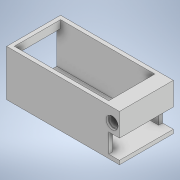
# Autodesk Inventor part: chaimber
Saved by Autodesk Inventor 2021 (Build 250183000, 183)
## iProperties
Created: 2024-03-14
Part Number: chaimber
Material: Generic
Document SubType Name: Modeling
Designer: 22hamfri
Density: 1 g/cm^3
Appearance: Default
Author: 22hamfri
Autodesk Inventor part; units mm, degrees
ref_plane "YZ Plane" through (0, 0, 0) normal (1, 0, 0) x (0, 1, 0)
ref_plane "XZ Plane" through (0, 0, 0) normal (0, 1, 0) x (-1, 0, 0)
ref_plane "XY Plane" through (0, 0, 0) normal (0, 0, 1) x (1, 0, 0)
sketch "Sketch1" plane through (0, 0, 0) normal (0, 1, 0) x (-1, 0, 0)
  line L0 (-24.5, 12) -> (24.5, 12)
  line L1 (24.5, 12) -> (24.5, -12)
  line L2 (24.5, -12) -> (-24.5, -12)
  line L3 (-24.5, -12) -> (-24.5, 12)
  line L4 (-24.5, 12) -> (24.5, -12) construction
  line L5 (24.5, 12) -> (-24.5, -12) construction
  line L6 (26.5, 14) -> (26.5, -14)
  line L7 (-24.5, 12) -> (-24.5, 14)
  line L8 (-24.5, 14) -> (26.5, 14)
  line L9 (26.5, -14) -> (-24.5, -14)
  line L10 (-24.5, -14) -> (-24.5, -12)
  line L11 (24.5, 12) -> (26.5, 12)
  line L12 (24.5, -12) -> (26.5, -12)
  point P0 (0, 0)
  dimension "d0" = 24
  dimension "d1" = 49
  dimension "d2" = 2
  dimension "d3" = 2
  dimension "d4" = 2
  constraints: 26 end point, 5 perpendicular, 2 horizontal, 2 midpoint, 2 parallel, 2 point on line, 2 vertical
  measures "d0" distance between parallel lines of L2 L0
  measures "d1" distance between parallel lines of L1 L3
  measures "d2" distance between parallel lines of L6 L1
  measures "d3" distance between parallel lines of L9 L2
  measures "d4" distance between parallel lines of L0 L8
extrude "Extrusion1" add sketch "Sketch1" against normal blind 2
extrude "Extrusion2" add sketch "Sketch1" along normal blind 22 contours L7 L8 L6 L11 L0 | L2 L12 L6 L9 L10
sketch "Sketch2" plane through (-26.5, 0, -12) normal (0, 0, 1) x (1, 0, 0)
  line L0 (0, 22) -> (0, 20)
  line L1 (0, 0) -> (0, 22) projected
  line L2 (0, 22) -> (2, 22)
  line L3 (0, 22) -> (51, 22) projected
  line L4 (2, 22) -> (2, 18)
  arc A0 (2, 18) -> (0, 20) centre (-3.1231, 14.8769) ccw
  line L5 (51, 0) -> (0, 0) projected
  point P0 (26.5, 0)
  dimension "d13" = 18
  dimension "d14" = 20
  dimension "d15" = 2
  dimension "d16" = 6
  constraints: 6 end point, 2 point on circle, 2 point on line, 1 centre point, 1 vertical
  measures "d13" distance from line of L5 L4.end
  measures "d14" distance from line of L5 L0.end
  measures "d15" distance between parallel lines of L1 L4
  measures "d16" radius of A0
extrude "Extrusion3" add sketch "Sketch2" along normal up to surface (24 mm away)
sketch "Sketch4" plane through (-26.5, -2, 14) normal (0, 0, 1) x (1, 0, 0)
  circle A0 centre (54.8, 17) radius 2.575
  circle A1 centre (54.8, 17) radius 3.1
  circle A2 centre (54.8, 17) radius 3.8
  line L0 (51, 2) -> (51, 24) projected
  line L1 (51, 12) -> (58.6, 12)
  line L2 (58.6, 12) -> (58.6, 24)
  line L3 (58.6, 24) -> (51, 24)
  point P0 (26.5, 2)
  dimension "d31" = 5.15
  dimension "d32" = 6.2
  dimension "d33" = 0.7
  dimension "d34" = 10
  dimension "d35" = 15
  constraints: 6 end point, 3 centre point, 3 perpendicular, 2 tangent, 1 point on line
  measures "d31" diameter of A0
  measures "d32" diameter of A1
  measures "d33" radial gap between concentric circles of A1 A2
  measures "d34" distance from line of L0.start L1
  measures "d35" vertical distance of L0.start A0.centre
extrude "Extrusion4" add sketch "Sketch4" against normal up to surface (28 mm away) contours A1 | A2 | L2 L1 L0 A2 | A2 L0 L3 L2
extrude "Extrusion5" cut sketch "Sketch4" against normal blind 1 contours A1
sketch "Sketch5" plane through (24.5, -2, 14) normal (1, 0, 0) x (0, 0, -1)
  line L0 (0, 0) -> (0, 12) projected
  line L1 (0, 2) -> (28, 2)
  line L2 (28, 0) -> (28, 12) projected
  line L3 (2, 2) -> (26, 2) projected
  line L4 (28, 12) -> (26, 12) projected
  line L5 (26, 2) -> (26, 12) projected
  line L6 (2, 2) -> (26, 2) projected
  line L7 (2, 12) -> (2, 2) projected
  line L8 (26, 12) -> (2, 12) projected
  line L9 (26, 12) -> (26, 24) projected
  line L10 (26, 24) -> (28, 24) projected
  line L11 (28, 24) -> (28, 12) projected
  line L12 (28, 12) -> (28, 0) projected
  line L13 (28, 0) -> (0, 0) projected
  line L14 (0, 0) -> (0, 12) projected
  line L15 (0, 12) -> (0, 24) projected
  line L16 (0, 24) -> (2, 24) projected
  line L17 (2, 24) -> (2, 12) projected
  line L18 (2, 12) -> (0, 12) projected
  line L19 (2, 24) -> (26, 24) projected
  point P0 (14, 2)
  constraints: 2 end point, 2 point on line, 1 collinear, 1 horizontal
extrude "Extrusion6" add sketch "Sketch5" along normal up to surface (7.6 mm away) contours L0 L1 L2 L13
sketch "Sketch6" plane through (-26.5, -2, -14) normal (0, 0, -1) x (-1, 0, 0)
  circle A0 centre (-54.8, 17) radius 3.1 projected
  circle A1 centre (-54.8, 17) radius 3.1 projected
  circle A2 centre (-54.8, 17) radius 2.575 projected
  circle A3 centre (-54.8, 17) radius 2.575 projected
  point P0 (-26.5, 2)
extrude "Extrusion7" cut sketch "Sketch6" against normal blind 1
extrude "Extrusion8" add sketch "Sketch5" along normal blind 2 contours L0 L18 L7 L1 | L1 L5 L4 L2
equation "\"d4\" = d3"
equation "\"d15\" = d2"
body "Solid1"
